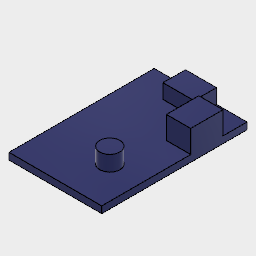
Powerboost 1000c v2 (Autodesk Fusion 360 design; units mm, degrees)
Autodesk Fusion 360 part; units mm, degrees
box "BoxPrimitive1" add length 36 width 23 height 1.7 placed x (0, 0, -1) y (-1, 0, 0) z (0, 1, 0) at (13, 0, 10)
sketch "Sketch5" plane through (0, 1.7, 0) normal (0, 1, 0) x (-1, 0, 0)
  line L0 (-13, -26) -> (10, -26)
  line L1 (10, -26) -> (10, 10)
  line L2 (10, 10) -> (-13, 10)
  line L3 (-13, 10) -> (-13, -26)
  line L4 (2.25, -26) -> (-5.45, -26)
  line L5 (-5.45, -26) -> (-5.45, -20.4)
  line L6 (-5.45, -20.4) -> (2.25, -20.4)
  line L7 (2.25, -20.4) -> (2.25, -26)
  dimension "d6" = 7.7
  dimension "d7" = 5.6
  dimension "d8" = 7.75
  constraint horizontal L4
  constraint vertical L5
  constraint horizontal L6
  constraint vertical L7
  constraint coincident L0
  measures "d8" distance of L1 L7
extrude "Extrude1" add sketch "Sketch5" along normal blind 3.6 contours L0 L4 L5 L6 L7
box "BoxPrimitive2" add length 8 width 6 height 5.6 placed x (0, 0, -1) y (-1, 0, 0) z (0, 1, 0) at (13, 1.7, -12.0226)
cylinder "CylinderPrimitive1" add diameter 5 height 3.8 placed x (1, 0, 0) y (0, 0, -1) z (0, 1, 0) at (5, 1.7, 0)
equation "d8 = 11.5 mm - 3.75 mm"
equation "d13 = 7.2 mm - 1.6 mm"
